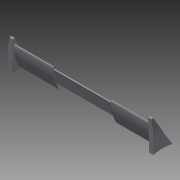
# Autodesk Inventor part: 2015 Front Spoiler 1
Saved by Autodesk Inventor 2015 (Build 190159000, 159)
## iProperties
Created: 2015-03-25
Part Number: 2015 Front Spoiler 1
Material: Generic
Document SubType Name: Modeling
Designer: Lks112201918
Density: 1 g/cm^3
Appearance: Default
Author: Lks112201918
Autodesk Inventor part; units mm, degrees
ref_plane "YZ Plane" through (0, 0, 0) normal (1, 0, 0) x (0, 1, 0)
ref_plane "XZ Plane" through (0, 0, 0) normal (0, 1, 0) x (-1, 0, 0)
ref_plane "XY Plane" through (0, 0, 0) normal (0, 0, 1) x (1, 0, 0)
sketch "Sketch1" plane through (0, 0, 0) normal (1, 0, 0) x (0, 1, 0)
  line L0 (0, 0) -> (0, -18)
  line L1 (0, -18) -> (10, -18)
  arc A0 (0, -18) -> (5, -17.3744) centre (5, -37.6672) ccw
  arc A1 (10, -18) -> (4.5107, -9) centre (113.0635, 51.0353) ccw
  arc A2 (4.5107, -9) -> (0, 0) centre (113.0635, 51.0353) ccw
  arc A3 (5, -17.3744) -> (10, -18) centre (5, -37.6672) ccw
  line L2 (0, -18) -> (0, 0)
  dimension "d0" = 18
  dimension "d1" = 10
  constraints: 12 point on circle, 6 end point, 4 centre point, 1 collinear, 1 concentric, 1 horizontal, 1 vertical
  measures "d0" distance of L0.start L0.end
  measures "d1" distance of L0.end L1.end
extrude "Extrusion1" add sketch "Sketch1" along normal blind 3 contours A1 A2 A0 A3 L0
sketch "Sketch2" plane through (0, 0, -18) normal (0, -1, 0) x (1, 0, 0)
  line L0 (0, 18) -> (0, 0) projected
  arc A0 (0, 0) -> (0, 8.2084) centre (59.4998, 4.1042) ccw
  line L1 (1.5, 18) -> (0, 18)
  line L2 (3, 18) -> (3, 0) projected
  line L3 (0, 18) -> (0, 8.2084)
  constraints: 4 end point, 3 point on circle, 2 perpendicular, 1 centre point, 1 point on line
extrude "Extrusion2" cut sketch "Sketch2" against normal through all contours L1 A0 L0
sketch "Sketch3" plane through (0, 0, -18) normal (0, -1, 0) x (1, 0, 0)
  arc A0 (2.5013, 11.9384) -> (3, 18) centre (138.3799, 3.8097) ccw
  arc A1 (2.5013, 11.9384) -> (3, 18) centre (138.3799, 3.8097) ccw
  line L0 (3, 18) -> (3, 0)
  line L1 (3, 18) -> (3, 0) projected
  line L2 (3, 0) -> (2.3116, 0)
  line L3 (0, 0) -> (3, 0) projected
  arc A2 (2.3116, 0) -> (2.5013, 11.9384) centre (138.3799, 3.8097) ccw
  point P0 (0, 18)
  constraints: 8 point on circle, 4 end point, 3 centre point, 1 collinear, 1 point on line
extrude "Extrusion3" cut sketch "Sketch3" against normal through all contours A2 L0 L2 A0
sketch "Sketch4" plane through (0, 0, 0) normal (-1, 0, 0) x (0, 0, 1)
  line L0 (0, 0) -> (-2.3228, 0)
  line L1 (-2.3228, 0) -> (-2.3228, 1.4083)
  line L2 (-2.3228, 1.4083) -> (0, 1.4083)
  line L3 (0, 1.4083) -> (0, 0)
  constraints: 8 end point, 2 parallel, 1 horizontal, 1 perpendicular
extrude "Extrusion4" cut sketch "Sketch4" against normal through all
sketch "Sketch5" plane through (0, 0, 0) normal (-1, 0, 0) x (0, 0, 1)
  spline S0 degree 3 poles (-5.2912, 1.3508) (-5.6719, 2.512) (-14.9331, 2.5632) (-17.0747, 4.0408) knots 0 0 0 0 1 1 1 1
  line L0 (-17.0747, 4.0408) -> (-16.7335, 3.4787) construction
  line L1 (-16.7335, 3.4787) -> (-11.5343, 1.3508) construction
  line L2 (-11.5343, 1.3508) -> (-7.961, 0.8289) construction
  line L3 (-7.961, 0.8289) -> (-5.5923, 0.7285) construction
  line L4 (-5.5923, 0.7285) -> (-5.1306, 0.9895) construction
  line L5 (-5.1306, 0.9895) -> (-5.2912, 1.3508) construction
  spline S1 degree 4 poles (-17.0747, 4.0408) (-16.7335, 3.4787) (-11.5343, 1.3508) (-7.961, 0.8289) (-5.5923, 0.7285) (-5.1306, 0.9895) (-5.2912, 1.3508) knots 1 1 1 1 1 2 3 4 4 4 4 4
  point P0 (0, 0)
  point P1 (-6.3741, 1.9135)
  point P2 (-12.4372, 2.8365)
  constraints: 7 other
extrude "Extrusion5" add sketch "Sketch5" against normal blind 23
sketch "Sketch6" plane through (0, 0, -18) normal (0, -1, 0) x (1, 0, 0)
  arc A0 (0, 8.2084) -> (0.9922, 15.6772) centre (59.4998, 4.1042) ccw
  line L0 (0.9922, 15.6772) -> (0, 15.6772)
  line L1 (0, 15.6772) -> (0, 8.2084)
  arc A1 (0, 0) -> (0, 8.2084) centre (59.4998, 4.1042) ccw
  point P0 (0, 18)
  constraints: 6 point on circle, 4 end point, 2 centre point, 1 horizontal, 1 perpendicular
extrude "Extrusion6" cut sketch "Sketch6" against normal through all contours L1 L0 A1
sketch "Sketch7" plane through (23, 0, 0) normal (1, 0, 0) x (0, 0, -1)
  line L0 (6.448, 1.0133) -> (12.9817, 2.2112)
  line L1 (12.9817, 2.2112) -> (12.8871, 2.727)
  line L2 (12.8871, 2.727) -> (6.3535, 1.5291)
  line L3 (6.3535, 1.5291) -> (6.448, 1.0133)
  point P0 (0, 0)
  constraints: 8 end point, 2 parallel, 1 perpendicular
extrude "Extrusion7" add sketch "Sketch7" along normal blind 15
mirror "Mirror1" about plane through (38, 1.8702, -9.6676) normal (1, 0, 0)
body "Solid1"
